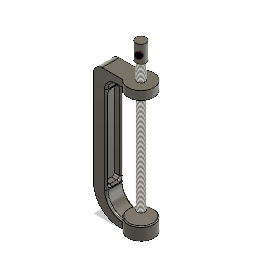
Graper (Autodesk Fusion 360 design; units mm, degrees)
Autodesk Fusion 360 part; units mm, degrees
sketch "Sketch1" plane through (0, 0, 0) normal (0, 0, 1) x (1, 0, 0)
  line L0 (0, 70) -> (15, 70)
  line L1 (15, 70) -> (15, -80)
  line L2 (15, -80) -> (0, -80)
  line L3 (0, -80) -> (0, 70)
  line L4 (15, 70) -> (45, 70)
  line L5 (45, 70) -> (45, 60)
  line L6 (45, 60) -> (15, 60)
  line L7 (15, 60) -> (15, 70)
  line L8 (15, -70.9267) -> (45, -70.9267)
  line L9 (45, -70.9267) -> (45, -80)
  line L10 (45, -80) -> (15, -80)
  line L11 (15, -80) -> (15, -70.9267)
  dimension "d1" = 150
  dimension "d4" = 30
  dimension "d5" = 30
  dimension "d44" = 0
  dimension "d45" = 0
  dimension "d46" = 0
  dimension "d47" = 0
  constraint horizontal L0
  constraint vertical L1
  constraint horizontal L2
  constraint vertical L3
  constraint horizontal L4
  constraint vertical L5
  constraint horizontal L6
  constraint vertical L7
  constraint horizontal L8
  constraint vertical L9
  constraint horizontal L10
  constraint vertical L11
  constraint coincident L1 L8.start
  measures "d1" distance of L0.start L2.end
  measures "d4" distance of L0.end L4.end
  measures "d5" distance of L8.start L8.end
extrude "Extrude1" add sketch "Sketch1" along normal blind 20 makes body 1
fillet "Fillet1" radius 10 1 edges at (0, 70, 10) on bodies 1
fillet "Fillet2" radius 10 1 edges at (15, 60, 10) on bodies 1
fillet "Fillet3" radius 30 1 edges at (0, -80, 10) on bodies 1
fillet "Fillet4" radius 20 1 edges at (15, -70.9267, 10) on bodies 1
sketch "Sketch3" plane through (0, -70.9267, 0) normal (0, 1, 0) x (-1, 0, 0)
  line L0 (-35, 0) -> (-35, 20)
  line L1 (-35, 20) -> (-45, 20)
  line L2 (-45, 20) -> (-45, 0)
  line L3 (-45, 0) -> (-35, 0)
  circle A0 centre (-45, 10) radius 15
  dimension "d10" = 30
  constraint midpoint L2 A0.centre
  measures "d10" diameter of A0
extrude "Extrude2" add sketch "Sketch3" along normal blind 5 and the other way blind 10 contours L0 L1 L2 L3 | A0 bodies 1
fillet "Fillet5" radius 1 1 edges at (58.9849, -65.9267, 4.5758) on bodies 1
sketch "Sketch4" plane through (0, 70, 0) normal (0, 1, 0) x (-1, 0, 0)
  line L0 (-10, 0) -> (-10, 20)
  line L1 (-10, 20) -> (-45, 20)
  line L2 (-45, 20) -> (-45, 0)
  line L3 (-45, 0) -> (-10, 0)
  circle A0 centre (-45, 10) radius 15
  circle A1 centre (-45, 10) radius 5
  point P0 (-30, 10)
  dimension "d16" = 10
  constraint midpoint L2 A0.centre
  constraint coincident A0 P0
  constraint concentric A0 A1
  measures "d16" diameter of A1
extrude "Extrude3" add sketch "Sketch4" against normal blind 10 contours L1 L2 L3 A0 A1 | L1 L2 L3 A0 A1 bodies 1
sketch "Sketch5" plane through (0, 70, 0) normal (0, 1, 0) x (-1, 0, 0)
  line L0 (-45, 15) -> (-45, 5)
  arc A0 (-45, 15) -> (-45, 5) centre (-45, 10) ccw
  arc A1 (-33.8197, 20) -> (-33.8197, 0) centre (-45, 10) ccw
  line L1 (-33.8197, 0) -> (-10, 0)
  line L2 (-10, 0) -> (-10, 20)
  line L3 (-10, 20) -> (-33.8197, 20)
  circle A2 centre (-45, 10) radius 5
  dimension "d19" = 10
  constraint concentric A0 A2
  measures "d19" diameter of A2
extrude "Extrude4" cut sketch "Sketch5" against normal blind 10 contours L0 A2 bodies 1
sketch "Sketch6" plane through (15, 0, 0) normal (1, 0, 0) x (0, 0, -1)
  line L0 (-20, -50.9267) -> (0, -50.9267)
  line L1 (0, -50.9267) -> (0, 50)
  line L2 (0, 50) -> (-20, 50)
  line L3 (-20, 50) -> (-20, -50.9267)
  line L4 (-17, 47) -> (-17, -47.9267)
  line L5 (-17, -47.9267) -> (-3, -47.9267)
  line L6 (-3, -47.9267) -> (-3, 47)
  line L7 (-3, 47) -> (-17, 47)
  dimension "d22" = 3
extrude "Extrude5" cut sketch "Sketch6" against normal blind 8 contours L4 L5 L6 L7 bodies 1
fillet "Fillet6" radius 3 1 edges at (11, 47, 3) on bodies 1
fillet "Fillet7" radius 3 1 edges at (11, 47, 17) on bodies 1
fillet "Fillet8" radius 3 2 edges at (11, -47.9267, 17) (11, -47.9267, 3) on bodies 1
fillet "Fillet9" radius 2 8 edges at (15, 46.1213, 16.1213) (15, 47, 10) (15, 46.1213, 3.8787) (15, -0.4634, 3) (15, -47.048, 3.8787) (15, -47.9267, 10) (15, -47.048, 16.1213) (15, -0.4634, 17) on bodies 1
fillet "Fillet10" radius 2 4 edges at (29.4098, 60, 0) (17.9289, 57.0711, 0) (15, -0.4634, 0) (20.4465, -64.6452, 0) on bodies 1
fillet "Fillet11" radius 2 4 edges at (20.4465, -64.6452, 20) (15, -0.4634, 20) (17.9289, 57.0711, 20) (29.4098, 60, 20) on bodies 1
thread "Thread1" "ISO Metric profile 10.0 M10x1.5 6H" major diameter 10.198 minor diameter 8.526 pitch 1.5 angle 60 resizes the face on face at (40.0062, 63.3333, 9.7508) on bodies 1
sketch "Sketch1 (2)" plane through (0, 70, 0) normal (0, 1, 0) x (-1, 0, 0) in component "Component"
  circle A0 centre (-45, 10) radius 4.263
  arc A1 (-33.8197, 20) -> (-33.8197, 0) centre (-45, 10) ccw
  line L0 (-33.8197, 0) -> (-10, 0)
  line L1 (-10, 0) -> (-10, 20)
  line L2 (-10, 20) -> (-33.8197, 20)
  dimension "d40" = 0
  dimension "d41" = 0
  dimension "d42" = 0
  dimension "d43" = 0
extrude "Extrude1'" add sketch "Sketch1 (2)" along normal blind 150 separate body contours A0 makes body 2 in component "Component"
thread "Thread1'" "ISO Metric profile 9.0 M9x1.25 6g" major diameter 8.866 minor diameter 7.4455 pitch 1.25 angle 60 resizes the face on face at (40.7423, 170, 9.7875) on bodies 2 in component "Component"
sketch "Sketch2" plane through (0, 220, 0) normal (0, 1, 0) x (-1, 0, 0) in component "Component"
  circle A0 centre (-45, 10) radius 4.433
  circle A1 centre (-45, 10) radius 6
  dimension "d33" = 12
  constraint concentric A0 A1
  measures "d33" diameter of A1
extrude "Extrude2'" add sketch "Sketch2" along normal blind 20 contours A0 | A1 bodies 2 in component "Component"
sketch "Sketch3 (2)" plane through (0, 220, 0) normal (0, -1, 0) x (1, 0, 0) in component "Component"
  circle A0 centre (45, 10) radius 6
  circle A1 centre (45, 10) radius 4.433
ref_plane "WorkPlane1" through (47.9137, 229.0846, 15.245) normal (0.485611, 0, 0.874175) x (-0.874175, 0, 0.485611) in component "Component"
sketch "Sketch4 (2)" plane through (47.9137, 229.0846, 15.245) normal (0.485611, 0, 0.874175) x (-0.874175, 0, 0.485611) in component "Component"
  circle A0 centre (0, 0) radius 2.5
  dimension "d37" = 5
  constraint coincident A0.centre origin
  measures "d37" diameter of A0
extrude "Extrude3'" cut sketch "Sketch4 (2)" against normal blind 15 bodies 2 in component "Component"
copy_body "Body->Comp1" bodies 1 removing the originals makes body 3 in component "Component'"
sketch "Sketch5 (2)" plane through (47.9137, 229.0846, 15.245) normal (0.485611, 0, 0.874175) x (-0.874175, 0, 0.485611) in component "Component"
extrude "Extrude4'" [suppressed] in component "Component"
component "Component" placed x (1, 0, 0) y (0, 1, 0) z (0, 0, 1) at (0, -130, 0)
component "Component'" placed x (1, 0, 0) y (0, 1, 0) z (0, 0, 1) at (0, 0, 0)
